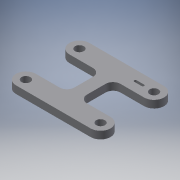
# Autodesk Inventor part: Base
Saved by Autodesk Inventor 2019 (Build 230136000, 136)
## iProperties
Created: 2021-07-19
Part Number: Base
Material: Типовые
Document SubType Name: Modeling
Designer: koryb
Density: 1 g/cm^3
Appearance: По умолчанию
Author: koryb
Autodesk Inventor part; units mm, degrees
ref_plane "YZ Plane" through (0, 0, 0) normal (1, 0, 0) x (0, 1, 0)
ref_plane "XZ Plane" through (0, 0, 0) normal (0, 1, 0) x (-1, 0, 0)
ref_plane "XY Plane" through (0, 0, 0) normal (0, 0, 1) x (1, 0, 0)
sketch "Эскиз1" plane through (0, 0, 0) normal (0, 1, 0) x (-1, 0, 0)
  circle A0 centre (15, 10.75) radius 1.75
  circle A1 centre (15, -10.75) radius 1.75
  circle A2 centre (-15, 10.75) radius 1.75
  circle A3 centre (-15, -10.75) radius 1.75
  line L0 (15, 10.75) -> (-15, 10.75) construction
  line L1 (15, 6.75) -> (-15, 6.75)
  line L2 (-15, 14.75) -> (15, 14.75)
  arc A4 (15, 6.75) -> (15, 14.75) centre (15, 10.75) ccw
  arc A5 (-15, 14.75) -> (-15, 6.75) centre (-15, 10.75) ccw
  line L3 (15, -10.75) -> (-15, -10.75) construction
  line L4 (15, -6.75) -> (-15, -6.75)
  line L5 (-15, -14.75) -> (15, -14.75)
  arc A6 (15, -14.75) -> (15, -6.75) centre (15, -10.75) ccw
  arc A7 (-15, -6.75) -> (-15, -14.75) centre (-15, -10.75) ccw
  line L6 (-2.5, -6.75) -> (2.5, -6.75)
  line L7 (2.5, -6.75) -> (2.5, 6.75)
  line L8 (2.5, 6.75) -> (-2.5, 6.75)
  line L9 (-2.5, 6.75) -> (-2.5, -6.75)
  line L10 (-2.5, -6.75) -> (2.5, 6.75) construction
  line L11 (2.5, -6.75) -> (-2.5, 6.75) construction
  point P0 (0, 0)
  point P1 (0, 10.75)
  point P2 (0, -10.75)
  dimension "d0" = 3.5
  dimension "d1" = 21.5
  dimension "d2" = 21.5
  dimension "d3" = 30
  dimension "d4" = 30
  dimension "d5" = 0
  dimension "d6" = 0
  dimension "d7" = 15
  dimension "d8" = 10.75
  dimension "d9" = 30
  dimension "d10" = 4
  dimension "d11" = 30
  dimension "d12" = 4
  dimension "d13" = 5
  constraints: 28 end point, 8 centre point, 8 point on circle, 8 tangent, 4 midpoint, 4 parallel, 3 equal radius, 3 horizontal, 2 coincident, 1 perpendicular, 1 point on line
  measures "d0" diameter of A0
  measures "d1" distance of A0.centre A1.centre
  measures "d2" distance of A3.centre A2.centre
  measures "d3" distance of A3.centre A1.centre
  measures "d4" distance of A2.centre A0.centre
  measures "d5" horizontal distance of A1.centre A0.centre
  measures "d6" vertical distance of A2.centre A0.centre
  measures "d7" horizontal distance of point (0, 0) A1.centre
  measures "d8" vertical distance of point (0, 0) A0.centre
  measures "d9" distance of L2.start L2.end
  measures "d10" radius of A4
  measures "d11" distance of L5.start L5.end
  measures "d12" radius of A6
  measures "d13" distance of L8.end L7.end
extrude "Выдавливание1" add sketch "Эскиз1" along normal blind 3
fillet "Сопряжение1" radius 3 4 edges at (-2.5, 1.5, -6.75) (-2.5, 1.5, 6.75) (2.5, 1.5, 6.75) (2.5, 1.5, -6.75)
sketch "Эскиз2" plane through (0, 3, 0) normal (0, 1, 0) x (1, 0, 0)
  line L0 (11, 10.75) -> (7, 10.75) construction
  line L1 (10.5, 11.25) -> (7.5, 11.25)
  line L2 (7.5, 10.25) -> (10.5, 10.25)
  arc A0 (10.5, 10.25) -> (10.5, 11.25) centre (10.5, 10.75) ccw
  arc A1 (7.5, 11.25) -> (7.5, 10.25) centre (7.5, 10.75) ccw
  point P0 (0, 0)
  point P1 (9, 10.75)
  point P2 (15, 10.75)
  dimension "d17" = 1
  dimension "d18" = 3
  dimension "d19" = 0
  dimension "d20" = 4
  constraints: 8 end point, 6 point on circle, 4 tangent, 2 centre point, 2 point on line, 1 horizontal, 1 midpoint, 1 parallel
  measures "d17" diameter of A1
  measures "d18" distance of L1.start L1.end
  measures "d19" vertical distance of point (9, 10.75) point (15, 10.75)
  measures "d20" distance of L0.start point (15, 10.75)
extrude "Выдавливание2" cut sketch "Эскиз2" against normal blind 3
